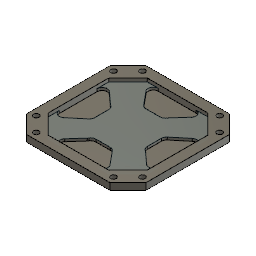
base v1 (Autodesk Fusion 360 design; units mm, degrees)
Autodesk Fusion 360 part; units mm, degrees
sketch "Sketch1" plane through (0, 0, 0) normal (0, 1, 0) x (1, 0, 0)
  line L0 (35, 35) -> (-35, 35)
  line L1 (-35, 35) -> (-35, -35)
  line L2 (-35, -35) -> (35, -35)
  line L3 (35, -35) -> (35, 35)
  line L4 (35, 35) -> (-35, -35) construction
  line L5 (-35, 35) -> (35, -35) construction
  line L6 (0, 0) -> (9.2688, 9.2688) construction
  line L7 (0, 0) -> (84.8528, 84.8528) construction
  line L8 (0, 0) -> (0, 35) construction
  line L9 (12.5, 35) -> (-12.5, 35)
  line L10 (-35, 12.5) -> (-35, -12.5)
  line L11 (-12.5, -35) -> (12.5, -35)
  line L12 (35, -12.5) -> (35, 12.5)
  line L13 (20.5061, 33.234) -> (33.234, 20.5061) construction
  line L14 (23.3345, 36.0624) -> (36.0624, 23.3345)
  line L15 (12.5, 35) -> (23.3345, 36.0624)
  line L16 (35, 12.5) -> (36.0624, 23.3345)
  circle A0 centre (22.6274, 31.1127) radius 1.6
  circle A1 centre (31.1127, 22.6274) radius 1.6
  line L17 (-35, 12.5) -> (-36.0624, 23.3345)
  line L18 (-36.0624, 23.3345) -> (-23.3345, 36.0624)
  line L19 (-12.5, 35) -> (-23.3345, 36.0624)
  circle A2 centre (-22.6274, 31.1127) radius 1.6
  circle A3 centre (-31.1127, 22.6274) radius 1.6
  line L20 (-12.5, -35) -> (-23.3345, -36.0624)
  line L21 (-23.3345, -36.0624) -> (-36.0624, -23.3345)
  line L22 (-35, -12.5) -> (-36.0624, -23.3345)
  circle A4 centre (-31.1127, -22.6274) radius 1.6
  circle A5 centre (-22.6274, -31.1127) radius 1.6
  line L23 (35, -12.5) -> (36.0624, -23.3345)
  line L24 (36.0624, -23.3345) -> (23.3345, -36.0624)
  line L25 (12.5, -35) -> (23.3345, -36.0624)
  circle A6 centre (22.6274, -31.1127) radius 1.6
  circle A7 centre (31.1127, -22.6274) radius 1.6
  dimension "d3" = 70
  dimension "d4" = 70
  dimension "d5" = 120
  dimension "d6" = 25
  dimension "d7" = 12.5
  dimension "d9" = 360
  dimension "d12" = 82
  dimension "d13" = 9
  dimension "d15" = 4
  dimension "d16" = 3.2
  dimension "d17" = 6
  dimension "d18" = 6
  dimension "d20" = 360
  constraint horizontal L0
  constraint perpendicular L0 L1
  constraint parallel L0 L2
  constraint parallel L1 L3
  constraint coincident L4 L6.start
  constraint coincident L5 L6.start
  constraint coincident L6.start L7.start
  constraint coincident L4 L6.end
  constraint perpendicular L5 L6
  constraint perpendicular L5 L7
  constraint midpoint L0 L8.end
  constraint coincident L0 L9.start
  constraint coincident L0 L9.end
  constraint parallel L0 L9
  constraint perpendicular L7 L13
  constraint perpendicular L7 L14
  constraint equal L13 L14
  constraint coincident L13 A0.centre
  constraint coincident L13 A1.centre
  constraint equal A0 A1
  measures "d3" distance of L1.end L2.end
  measures "d4" distance of L0.end L1.end
  measures "d5" distance of L6.start L7.end
  measures "d6" distance of L9.start L9.end
  measures "d7" distance of L8 L9.end
  measures "d12" distance of L7.end L13
  measures "d13" distance of L4 L14.end
  measures "d15" distance of L13.end L14.end
  measures "d16" diameter of A0
  measures "d17" distance of L7 A0.centre
  measures "d18" distance of L7 A1.centre
extrude "Extrude1" add sketch "Sketch1" along normal blind 4 contours L0 L1 L2 L3 L9 L10 L11 L12 L14 L18 L21 L24
sketch "Sketch2" plane through (0, 4, 0) normal (0, 1, 0) x (-1, 0, 0)
  circle A0 centre (-22.6274, 31.1127) radius 1.6
  circle A1 centre (-31.1127, 22.6274) radius 1.6
  circle A2 centre (31.1127, -22.6274) radius 1.6
  circle A3 centre (31.1127, 22.6274) radius 1.6
  circle A4 centre (22.6274, 31.1127) radius 1.6
  circle A5 centre (22.6274, -31.1127) radius 1.6
  circle A6 centre (-31.1127, -22.6274) radius 1.6
  circle A7 centre (-22.6274, -31.1127) radius 1.6
  line L0 (24.397, 35) -> (-24.397, 35)
  line L1 (-24.397, 35) -> (-35, 24.397)
  line L2 (-35, 24.397) -> (-35, -24.397)
  line L3 (-35, -24.397) -> (-24.397, -35)
  line L4 (-24.397, -35) -> (24.397, -35)
  line L5 (24.397, -35) -> (35, -24.397)
  line L6 (35, -24.397) -> (35, 24.397)
  line L7 (35, 24.397) -> (24.397, 35)
  line L8 (0, 0) -> (0, -35) construction
  line L9 (0, 0) -> (35, 0) construction
  line L10 (17.669, -29) -> (-17.669, -29)
  line L11 (-17.669, -29) -> (-29, -17.669)
  line L12 (-29, -17.669) -> (-29, 17.669)
  line L13 (-29, 17.669) -> (-17.669, 29)
  line L14 (-17.669, 29) -> (17.669, 29)
  line L15 (17.669, 29) -> (29, 17.669)
  line L16 (29, 17.669) -> (29, -17.669)
  line L17 (29, -17.669) -> (17.669, -29)
  dimension "d23" = 6
  dimension "d24" = 6
  dimension "d25" = 9
  dimension "d26" = 9
  constraint coincident L8.start L9.start
  constraint midpoint L4 L8.end
  constraint midpoint L6 L9.end
  constraint perpendicular L8 L10
  constraint parallel L8 L12
  constraint perpendicular L11 L13
  constraint perpendicular L12 L14
  constraint perpendicular L9 L16
  constraint equal L10 L16
  constraint equal L14 L16
  constraint equal L12 L14
  constraint equal L11 L17
  constraint equal L11 L13
  constraint equal L13 L15
  constraint parallel L7 L15
  measures "d23" distance of L6 L16
  measures "d24" distance of L0 L14
  measures "d25" distance of L7 L15
  measures "d26" distance of L3 L11
extrude "Extrude2" cut sketch "Sketch2" against normal blind 2 contours L10 L11 L12 L13 L14 L15 L16 L17
sketch "Sketch3" plane through (0, 2, 0) normal (0, 1, 0) x (-1, 0, 0)
  line L0 (29, -17.669) -> (29, 17.669)
  line L1 (29, 17.669) -> (17.669, 29)
  line L2 (17.669, 29) -> (-17.669, 29)
  line L3 (-17.669, 29) -> (-29, 17.669)
  line L4 (-29, 17.669) -> (-29, -17.669)
  line L5 (-29, -17.669) -> (-17.669, -29)
  line L6 (-17.669, -29) -> (17.669, -29)
  line L7 (17.669, -29) -> (29, -17.669)
  line L8 (0, 0) -> (0, -29) construction
  line L9 (0, 0) -> (29, 0) construction
  line L10 (15, -3.7839) -> (15, 4.5951)
  line L11 (16.0792, 6.8995) -> (24.0792, 13.5676)
  line L12 (15, -6) -> (15.0349, -6)
  line L13 (17.0557, -6.7828) -> (23.9792, -13.0929)
  line L14 (29, -10.8757) -> (29, 11.2631)
  arc A0 (23.9792, -13.0929) -> (29, -10.8757) centre (26, -10.8757) ccw
  arc A1 (29, 11.2631) -> (24.0792, 13.5676) centre (26, 11.2631) ccw
  arc A2 (16.0792, 6.8995) -> (15, 4.5951) centre (18, 4.5951) ccw
  arc A3 (17.0557, -6.7828) -> (16.5174, -6.3919) centre (15.0349, -9) ccw
  arc A4 (15, -3.7839) -> (16.5174, -6.3919) centre (18, -3.7839) ccw
  arc A5 (13.0929, 23.9792) -> (10.8757, 29) centre (10.8757, 26) ccw
  line L15 (10.8757, 29) -> (-11.2631, 29)
  line L16 (6.7828, 17.0557) -> (13.0929, 23.9792)
  arc A6 (-11.2631, 29) -> (-13.5676, 24.0792) centre (-11.2631, 26) ccw
  line L17 (-6.8995, 16.0792) -> (-13.5676, 24.0792)
  arc A7 (-6.8995, 16.0792) -> (-4.5951, 15) centre (-4.5951, 18) ccw
  line L18 (3.7839, 15) -> (-4.5951, 15)
  arc A8 (3.7839, 15) -> (6.3919, 16.5174) centre (3.7839, 18) ccw
  arc A9 (-23.9792, 13.0929) -> (-29, 10.8757) centre (-26, 10.8757) ccw
  line L19 (-29, 10.8757) -> (-29, -11.2631)
  line L20 (-17.0557, 6.7828) -> (-23.9792, 13.0929)
  arc A10 (-29, -11.2631) -> (-24.0792, -13.5676) centre (-26, -11.2631) ccw
  line L21 (-16.0792, -6.8995) -> (-24.0792, -13.5676)
  arc A11 (-16.0792, -6.8995) -> (-15, -4.5951) centre (-18, -4.5951) ccw
  line L22 (-15, 3.7839) -> (-15, -4.5951)
  arc A12 (-15, 3.7839) -> (-16.5174, 6.3919) centre (-18, 3.7839) ccw
  arc A13 (-13.0929, -23.9792) -> (-10.8757, -29) centre (-10.8757, -26) ccw
  line L23 (-10.8757, -29) -> (11.2631, -29)
  line L24 (-6.7828, -17.0557) -> (-13.0929, -23.9792)
  arc A14 (11.2631, -29) -> (13.5676, -24.0792) centre (11.2631, -26) ccw
  line L25 (6.8995, -16.0792) -> (13.5676, -24.0792)
  arc A15 (6.8995, -16.0792) -> (4.5951, -15) centre (4.5951, -18) ccw
  line L26 (-3.7839, -15) -> (4.5951, -15)
  arc A16 (-3.7839, -15) -> (-6.3919, -16.5174) centre (-3.7839, -18) ccw
  line L27 (10.8757, 29) -> (-11.2631, 29)
  point P0 (15, 6)
  dimension "d29" = 15
  dimension "d30" = 12
  dimension "d31" = 6
  dimension "d32" = 3
  dimension "d34" = 360
  constraint coincident L8.start L9.start
  constraint midpoint L6 L8.end
  constraint midpoint L0 L9.end
  constraint perpendicular L9 L10
  constraint perpendicular L10 L12
  constraint tangent L13 A0
  constraint tangent L14 A0
  constraint tangent L11 A1
  constraint tangent L14 A1
  constraint equal A0 A1
  constraint coincident P0 L10
  constraint coincident P0 L11
  constraint tangent L10 A2
  constraint tangent L11 A2
  constraint equal A0 A2
  constraint tangent L12 A3
  constraint tangent L13 A3
  constraint equal A0 A3
  constraint tangent L10 A4
  constraint tangent A3 A4
  constraint equal A0 A4
  measures "d29" distance of L8.start L10
  measures "d30" distance of L12.start P0
  measures "d31" distance of L9 P0
  measures "d32" radius of A0
extrude "Extrude3" cut sketch "Sketch3" against normal blind 1.5 contours L0 L10 L11 L13 L14 A0 A1 A2 A3 A4
pattern_circular "C-Pattern1" count 4 over 360 about axis through (0, 1.75, 0) along (0, 1, 0) of "Extrude3"
sketch "Sketch4" plane through (0, 2, 0) normal (0, 1, 0) x (-1, 0, 0)
  arc A0 (-13.0929, -23.9792) -> (-10.8757, -29) centre (-10.8757, -26) ccw
  line L0 (-13.0929, -23.9792) -> (-6.7828, -17.0557)
  arc A1 (-6.7828, -17.0557) -> (-6.3919, -16.5174) centre (-9, -15.0349) ccw
  arc A2 (-3.7839, -15) -> (-6.3919, -16.5174) centre (-3.7839, -18) ccw
  line L1 (-3.7839, -15) -> (4.5951, -15)
  arc A3 (6.8995, -16.0792) -> (4.5951, -15) centre (4.5951, -18) ccw
  line L2 (6.8995, -16.0792) -> (13.5676, -24.0792)
  arc A4 (11.2631, -29) -> (13.5676, -24.0792) centre (11.2631, -26) ccw
  line L3 (11.2631, -29) -> (17.669, -29)
  line L4 (17.669, -29) -> (29, -17.669)
  line L5 (29, -17.669) -> (29, -10.8757)
  arc A5 (23.9792, -13.0929) -> (29, -10.8757) centre (26, -10.8757) ccw
  line L6 (23.9792, -13.0929) -> (17.0557, -6.7828)
  arc A6 (17.0557, -6.7828) -> (16.5174, -6.3919) centre (15.0349, -9) ccw
  arc A7 (15, -3.7839) -> (16.5174, -6.3919) centre (18, -3.7839) ccw
  line L7 (15, -3.7839) -> (15, 4.5951)
  arc A8 (16.0792, 6.8995) -> (15, 4.5951) centre (18, 4.5951) ccw
  line L8 (16.0792, 6.8995) -> (24.0792, 13.5676)
  arc A9 (29, 11.2631) -> (24.0792, 13.5676) centre (26, 11.2631) ccw
  line L9 (29, 11.2631) -> (29, 17.669)
  line L10 (29, 17.669) -> (17.669, 29)
  line L11 (17.669, 29) -> (10.8757, 29)
  arc A10 (13.0929, 23.9792) -> (10.8757, 29) centre (10.8757, 26) ccw
  line L12 (13.0929, 23.9792) -> (6.7828, 17.0557)
  arc A11 (6.7828, 17.0557) -> (6.3919, 16.5174) centre (9, 15.0349) ccw
  arc A12 (3.7839, 15) -> (6.3919, 16.5174) centre (3.7839, 18) ccw
  line L13 (3.7839, 15) -> (-4.5951, 15)
  arc A13 (-6.8995, 16.0792) -> (-4.5951, 15) centre (-4.5951, 18) ccw
  line L14 (-6.8995, 16.0792) -> (-13.5676, 24.0792)
  arc A14 (-11.2631, 29) -> (-13.5676, 24.0792) centre (-11.2631, 26) ccw
  line L15 (-11.2631, 29) -> (-17.669, 29)
  line L16 (-17.669, 29) -> (-29, 17.669)
  line L17 (-29, 17.669) -> (-29, 10.8757)
  arc A15 (-23.9792, 13.0929) -> (-29, 10.8757) centre (-26, 10.8757) ccw
  line L18 (-23.9792, 13.0929) -> (-17.0557, 6.7828)
  arc A16 (-17.0557, 6.7828) -> (-16.5174, 6.3919) centre (-15.0349, 9) ccw
  arc A17 (-15, 3.7839) -> (-16.5174, 6.3919) centre (-18, 3.7839) ccw
  line L19 (-15, 3.7839) -> (-15, -4.5951)
  arc A18 (-16.0792, -6.8995) -> (-15, -4.5951) centre (-18, -4.5951) ccw
  line L20 (-16.0792, -6.8995) -> (-24.0792, -13.5676)
  arc A19 (-29, -11.2631) -> (-24.0792, -13.5676) centre (-26, -11.2631) ccw
  line L21 (-29, -11.2631) -> (-29, -17.669)
  line L22 (-29, -17.669) -> (-17.669, -29)
  line L23 (-17.669, -29) -> (-10.8757, -29)
